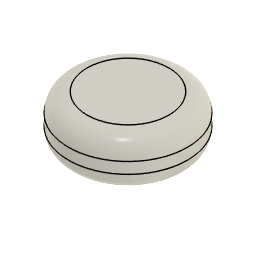
Front Wheel (Autodesk Fusion 360 design; units mm, degrees)
Autodesk Fusion 360 part; units mm, degrees
sketch "スケッチ1" plane through (0, 0, 0) normal (0, 0, 1) x (1, 0, 0)
  circle A0 centre (0, 0) radius 16
  dimension "d1" = 32
  constraint coincident A0.centre origin
  measures "d1" diameter of A0
extrude "押し出し1" add sketch "スケッチ1" along normal blind 13
fillet "フィレット1" radius 5 2 edges at (-14.9172, -5.7858, 0) (-14.9172, -5.7858, 13)
sketch "スケッチ2" plane through (0, 0, 0) normal (0, 0, -1) x (1, 0, 0)
  circle A0 centre (0, 0) radius 11
  circle A1 centre (0, 0) radius 3
  circle A2 centre (0, 0) radius 1.05
  dimension "d6" = 6
  dimension "d7" = 2.1
  constraint coincident A0.centre A1.centre
  measures "d6" diameter of A1
  measures "d7" diameter of A2
extrude "押し出し2" add sketch "スケッチ2" along normal blind 4 contours A1
